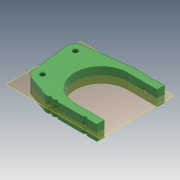
# Autodesk Inventor part: bloco-dedo-1
Saved by Autodesk Inventor 2017 (Build 210142000, 142)
## iProperties
Created: 2018-05-30
Part Number: bloco-dedo-1
Material: Generic
Document SubType Name: Modeling
Designer: Luiz Gustavo
Density: 1 g/cm^3
Appearance: Smooth - Dark Forest Green
Mass: 12.4241 g
Surface Area: 57.8047 cm^2
Volume: 12.4241 cm^3
Author: Luiz Gustavo
Autodesk Inventor part; units mm, degrees
ref_plane "YZ Plane" through (0, 0, 0) normal (1, 0, 0) x (0, 1, 0)
ref_plane "XZ Plane" through (0, 0, 0) normal (0, 1, 0) x (-1, 0, 0)
ref_plane "XY Plane" through (0, 0, 0) normal (0, 0, 1) x (1, 0, 0)
sketch "Sketch1" plane through (0, 0, 0) normal (0, 0, 1) x (1, 0, 0)
  line L0 (40, 15) -> (40, 0) construction
  circle A0 centre (-2.6718, 25) radius 1.55
  circle A1 centre (0, 0) radius 1.55
  arc A2 (2.1334, 28.593) -> (-3.4383, 30.9508) centre (-2.6718, 25) ccw construction
  arc A3 (-5.966, -0.6376) -> (-2.0133, -5.6521) centre (0, 0) ccw
  line L1 (-8.6378, 24.3624) -> (-5.966, -0.6376)
  line L2 (0, -6) -> (28, -6) construction
  line L3 (40, 0) -> (48, 0) construction
  line L4 (48, 0) -> (48, -6) construction
  line L5 (48, -6) -> (48, -11)
  line L6 (48, -11) -> (41.3764, -11)
  line L7 (13, -11) -> (-2.0133, -5.6521)
  line L8 (28, -6) -> (48, -6)
  line L9 (28, 30) -> (48, 30)
  line L10 (48, 30) -> (48, 35)
  line L11 (48, 35) -> (41.3764, 35)
  line L12 (48, -6) -> (48, 30) construction
  arc A4 (-8.6378, 24.3624) -> (2.1334, 28.593) centre (-2.6718, 25) ccw construction
  arc A5 (0, -6) -> (-5.966, -0.6376) centre (0, 0) ccw construction
  line L13 (28, -6) -> (28, 30) construction
  line L14 (28, 35) -> (-3.4383, 30.9508)
  arc A6 (-3.4383, 30.9508) -> (-8.6378, 24.3624) centre (-2.6718, 25) ccw
  line L15 (28, 35) -> (28, 30) construction
  arc A7 (28, 30) -> (28, -6) centre (28, 12) ccw
  line L16 (40, 15) -> (40, 35) construction
  line L17 (38.6236, 35) -> (40, 34)
  line L18 (40, 34) -> (41.3764, 35)
  line L19 (38.6236, 35) -> (41.3764, 35) construction
  line L20 (40, 34) -> (40, 35) construction
  line L21 (41.3764, -11) -> (40, -10)
  line L22 (40, -10) -> (38.6236, -11)
  line L23 (41.3764, -11) -> (38.6236, -11) construction
  line L24 (40, -10) -> (40, -11) construction
  line L25 (40, 0) -> (40, -11) construction
  line L26 (21.5514, -11) -> (20.175, -10)
  line L27 (20.175, -10) -> (18.7986, -11)
  line L28 (20.175, -10) -> (20.175, -11) construction
  line L29 (20.175, -10) -> (40, -10) construction
  line L30 (17.5514, -11) -> (16.175, -10)
  line L31 (16.175, -10) -> (14.7986, -11)
  line L32 (16.175, -10) -> (20.175, -10) construction
  line L33 (16.175, -10) -> (16.175, -11) construction
  line L34 (14.7986, -11) -> (13, -11)
  line L35 (17.5514, -11) -> (14.7986, -11) construction
  line L36 (21.5514, -11) -> (38.6236, -11)
  line L37 (17.5514, -11) -> (18.7986, -11)
  line L38 (18.7986, -11) -> (21.5514, -11) construction
  line L39 (38.6236, 35) -> (28, 35)
  line L40 (41.3764, 35) -> (38.6236, 35) construction
  arc A8 (-2.0133, -5.6521) -> (0, -6) centre (0, 0) ccw construction
  dimension "d0" = 3.1
  dimension "d1" = 12
  dimension "d4" = 5
  dimension "d6" = 15
  dimension "d7" = 36
  dimension "d40" = 108
  dimension "d41" = 1
  dimension "d42" = 108
  dimension "d43" = 1
  dimension "d46" = 108
  dimension "d48" = 19.825
  dimension "d49" = 108
  dimension "d51" = 4
  dimension "d52" = 12
  dimension "d53" = 8
  constraints: 80 end point, 19 perpendicular, 14 point on circle, 12 tangent, 9 centre point, 9 horizontal, 5 midpoint, 4 coincident, 4 vertical, 3 equal length, 2 equal radius, 2 point on line, 1 parallel, 1 symmetric about line
  measures "d0" diameter of A0
  measures "d1" diameter of A2
  measures "d4" distance of L4.end L5.end
  measures "d6" horizontal distance of L7.start L2.end
  measures "d7" distance between parallel lines of L8 L9
  measures "d40" angle of L17 L18
  measures "d41" distance of L16.end L17.end
  measures "d42" angle of L21 L22
  measures "d43" distance of L24.end L21.end
  measures "d46" angle of L26 L27
  measures "d48" distance of L26.end L21.end
  measures "d49" angle of L30 L31
  measures "d51" distance of L30.end L26.end
  measures "d52" distance between parallel lines of L13 L25
  measures "d53" distance between parallel lines of L25 L5
extrude "Extrusion1" add sketch "Sketch1" along normal mid plane 10
ref_plane "Work Plane1" through (0, 0, 0) normal (0, 0, 1) x (1, 0, 0)
sketch "Sketch4" plane through (0, 0, 0) normal (0, 1, 0) x (-1, 0, 0)
  line L0 (-40, -5) -> (-40, 5) projected
  line L1 (-20.175, -5) -> (-20.175, 5) projected
  line L2 (-14.7986, -5) -> (-14.7986, 5) projected
  circle A0 centre (-40, 0) radius 1.5
  circle A1 centre (-20.175, 0) radius 1.25
  circle A2 centre (-14.7986, 0) radius 1.25
  point P0 (0, 0)
  dimension "d55" = 3
  dimension "d56" = 2.5
  constraints: 3 centre point, 3 coincident, 3 midpoint, 1 equal radius
  measures "d55" diameter of A0
  measures "d56" diameter of A1
extrude "Extrusion4" cut sketch "Sketch4" against normal through all contours A1 L1 | L1 A1 | A2 L2 | L2 A2
extrude "Extrusion5" cut sketch "Sketch4" along normal through all both and the other way through all contours A0 L0 | L0 A0
chamfer "Chamfer1" [suppressed]
equation "\"d46\" = d42"
equation "\"d49\" = d50"
equation "\"d50\" = 108deg"
body "Solid1"
